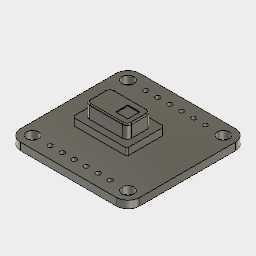
3538 AMG8833 IR Thermal Camera (Autodesk Fusion 360 design; units mm, degrees)
Autodesk Fusion 360 part; units mm, degrees
sketch "AMG8833_REV-B" plane through (0, 0, 0) normal (0, 0, 1) x (1, 0, 0)
  arc A0 (2.54, 25.4) -> (0, 22.86) centre (2.54, 22.86) ccw
  line L0 (2.54, 25.4) -> (22.86, 25.4)
  line L1 (22.86, 0) -> (2.54, 0)
  arc A1 (0, 2.54) -> (2.54, 0) centre (2.54, 2.54) ccw
  line L2 (0, 2.54) -> (0, 22.86)
  arc A2 (22.86, 0) -> (25.4, 2.54) centre (22.86, 2.54) ccw
  arc A3 (25.4, 22.86) -> (22.86, 25.4) centre (22.86, 22.86) ccw
  line L3 (25.4, 22.86) -> (25.4, 2.54)
  circle A4 centre (2.54, 22.86) radius 1.758
  circle A5 centre (8.89, 2.54) radius 0.889
  circle A6 centre (2.54, 22.86) radius 1.758
  circle A7 centre (11.43, 2.54) radius 0.889
  circle A8 centre (22.86, 22.86) radius 1.758
  circle A9 centre (22.86, 2.54) radius 1.758
  circle A10 centre (6.35, 2.54) radius 0.889
  circle A11 centre (22.86, 2.54) radius 1.758
  circle A12 centre (11.43, 2.54) radius 0.889
  circle A13 centre (16.51, 22.86) radius 0.889
  circle A14 centre (13.97, 22.86) radius 0.889
  circle A15 centre (6.35, 22.86) radius 0.889
  circle A16 centre (6.35, 22.86) radius 0.889
  circle A17 centre (2.54, 2.54) radius 1.758
  circle A18 centre (19.05, 22.86) radius 0.889
  circle A19 centre (8.89, 22.86) radius 0.889
  circle A20 centre (11.43, 22.86) radius 0.889
  circle A21 centre (11.43, 22.86) radius 0.889
  circle A22 centre (13.97, 2.54) radius 0.889
  circle A23 centre (16.51, 2.54) radius 0.889
  circle A24 centre (16.51, 2.54) radius 0.889
  circle A25 centre (19.05, 22.86) radius 0.889
  circle A26 centre (16.51, 22.86) radius 0.889
  circle A27 centre (13.97, 22.86) radius 0.889
  circle A28 centre (8.89, 22.86) radius 0.889
  circle A29 centre (6.35, 2.54) radius 0.889
  circle A30 centre (19.05, 2.54) radius 0.889
  circle A31 centre (8.89, 2.54) radius 0.889
  circle A32 centre (13.97, 2.54) radius 0.889
  circle A33 centre (22.86, 22.86) radius 1.758
  circle A34 centre (2.54, 2.54) radius 1.758
  circle A35 centre (19.05, 2.54) radius 0.889
extrude "Extrude2" add sketch "AMG8833_REV-B" along normal blind 1.6
sketch "holes" plane through (0, 0, 1.6) normal (0, 0, 1) x (-1, 0, 0)
  circle A0 centre (-19.05, -2.54) radius 0.889
  circle A1 centre (-6.35, -22.86) radius 0.889
  circle A2 centre (-2.54, -2.54) radius 1.758
  circle A3 centre (-13.97, -22.86) radius 0.889
  circle A4 centre (-19.05, -22.86) radius 0.889
  circle A5 centre (-22.86, -2.54) radius 1.758
  circle A6 centre (-22.86, -22.86) radius 1.758
  circle A7 centre (-6.35, -2.54) radius 0.889
  circle A8 centre (-16.51, -2.54) radius 0.889
  circle A9 centre (-2.54, -22.86) radius 1.758
  circle A10 centre (-13.97, -2.54) radius 0.889
  circle A11 centre (-8.89, -2.54) radius 0.889
  circle A12 centre (-8.89, -22.86) radius 0.889
  circle A13 centre (-11.43, -22.86) radius 0.889
  circle A14 centre (-11.43, -2.54) radius 0.889
  circle A15 centre (-16.51, -22.86) radius 0.889
  arc A16 (-2.54, -25.4) -> (0, -22.86) centre (-2.54, -22.86) ccw
  line L0 (0, -22.86) -> (0, -2.54)
  arc A17 (0, -2.54) -> (-2.54, 0) centre (-2.54, -2.54) ccw
  line L1 (-2.54, 0) -> (-22.86, 0)
  arc A18 (-22.86, 0) -> (-25.4, -2.54) centre (-22.86, -2.54) ccw
  line L2 (-25.4, -2.54) -> (-25.4, -22.86)
  arc A19 (-25.4, -22.86) -> (-22.86, -25.4) centre (-22.86, -22.86) ccw
  line L3 (-22.86, -25.4) -> (-2.54, -25.4)
  circle A20 centre (-22.86, -22.86) radius 1.27
  circle A21 centre (-2.54, -22.86) radius 1.27
  circle A22 centre (-2.54, -2.54) radius 1.27
  circle A23 centre (-22.86, -2.54) radius 1.27
  circle A24 centre (-19.05, -2.54) radius 0.5
  circle A25 centre (-16.51, -2.54) radius 0.5
  circle A26 centre (-13.97, -2.54) radius 0.5
  circle A27 centre (-11.43, -2.54) radius 0.5
  circle A28 centre (-8.89, -2.54) radius 0.5
  circle A29 centre (-6.35, -2.54) radius 0.5
  circle A30 centre (-19.05, -22.86) radius 0.5
  circle A31 centre (-16.51, -22.86) radius 0.5
  circle A32 centre (-13.97, -22.86) radius 0.5
  circle A33 centre (-11.43, -22.86) radius 0.5
  circle A34 centre (-8.89, -22.86) radius 0.5
  circle A35 centre (-6.35, -22.86) radius 0.5
  dimension "d5" = 2.54
  dimension "d6" = 2.54
  dimension "d7" = 2.54
  dimension "d8" = 2.54
  dimension "d9" = 1
  dimension "d15" = 2.54
  dimension "d16" = 0
  dimension "d17" = 1
  dimension "d20" = 2.54
  dimension "d21" = 0
  measures "d5" diameter of A20
  measures "d6" diameter of A21
  measures "d7" diameter of A22
  measures "d8" diameter of A23
  measures "d9" diameter of A24
  measures "d17" diameter of A30
extrude "Extrude3" add sketch "holes" against normal blind 1.6 contours A0 | A1 | A2 | A3 | A4 | A5 | A6 | A7 | A8 | A9 | A10 | A11 | A12 | A13 | A14 | A15
sketch "lens base" plane through (0, 0, 1.6) normal (0, 0, 1) x (-1, 0, 0)
  circle A0 centre (-22.86, -2.54) radius 1.27
  circle A1 centre (-11.43, -2.54) radius 0.5
  circle A2 centre (-22.86, -22.86) radius 1.27
  circle A3 centre (-11.43, -22.86) radius 0.5
  circle A4 centre (-2.54, -22.86) radius 1.27
  circle A5 centre (-13.97, -22.86) radius 0.5
  circle A6 centre (-2.54, -2.54) radius 1.27
  circle A7 centre (-13.97, -2.54) radius 0.5
  circle A8 centre (-19.05, -2.54) radius 0.5
  circle A9 centre (-8.89, -2.54) radius 0.5
  circle A10 centre (-19.05, -22.86) radius 0.5
  circle A11 centre (-8.89, -22.86) radius 0.5
  circle A12 centre (-6.35, -22.86) radius 0.5
  circle A13 centre (-16.51, -22.86) radius 0.5
  circle A14 centre (-6.35, -2.54) radius 0.5
  circle A15 centre (-16.51, -2.54) radius 0.5
  arc A16 (-2.54, -25.4) -> (0, -22.86) centre (-2.54, -22.86) ccw
  line L0 (0, -22.86) -> (0, -2.54)
  arc A17 (0, -2.54) -> (-2.54, 0) centre (-2.54, -2.54) ccw
  line L1 (-2.54, 0) -> (-22.86, 0)
  arc A18 (-22.86, 0) -> (-25.4, -2.54) centre (-22.86, -2.54) ccw
  line L2 (-25.4, -2.54) -> (-25.4, -22.86)
  arc A19 (-25.4, -22.86) -> (-22.86, -25.4) centre (-22.86, -22.86) ccw
  line L3 (-22.86, -25.4) -> (-2.54, -25.4)
  line L4 (-4.868, -16.7) -> (-16.468, -16.7)
  line L5 (-16.468, -16.7) -> (-16.468, -8.7)
  line L6 (-16.468, -8.7) -> (-4.868, -8.7)
  line L7 (-4.868, -8.7) -> (-4.868, -16.7)
  line L8 (-10.668, -16.7) -> (-10.668, -8.7) construction
  line L9 (-16.468, -12.7) -> (-4.868, -12.7) construction
  dimension "d24" = 11.6
  dimension "d25" = 8
  dimension "d26" = 10.668
  dimension "d27" = 12.7
  measures "d24" distance of L4.start L4.end
  measures "d25" distance of L4.start L6.end
  measures "d26" distance of L0 L8
  measures "d27" distance of L1 L9
extrude "Extrude4" add sketch "lens base" along normal blind 1.5 contours L4 L5 L6 L7
sketch "lens" plane through (0, 0, 3.1) normal (0, 0, 1) x (-1, 0, 0)
  line L0 (-4.868, -8.7) -> (-16.468, -8.7)
  line L1 (-16.468, -8.7) -> (-16.468, -16.7)
  line L2 (-16.468, -16.7) -> (-4.868, -16.7)
  line L3 (-4.868, -16.7) -> (-4.868, -8.7)
  line L4 (-11.368, -14) -> (-13.968, -14)
  line L5 (-13.968, -14) -> (-13.968, -11.4)
  line L6 (-13.968, -11.4) -> (-11.368, -11.4)
  line L7 (-11.368, -11.4) -> (-11.368, -14)
  line L8 (-11.368, -12.7) -> (-13.968, -12.7) construction
  line L9 (-12.668, -14) -> (-12.668, -11.4) construction
  line L10 (-10.668, -16.7) -> (-10.668, -8.7) construction
  line L11 (-4.868, -12.7) -> (-16.468, -12.7) construction
  line L12 (-6.218, -15.35) -> (-15.118, -15.35)
  line L13 (-15.118, -15.35) -> (-15.118, -10.05)
  line L14 (-15.118, -10.05) -> (-6.218, -10.05)
  line L15 (-6.218, -10.05) -> (-6.218, -15.35)
  line L16 (-10.668, -15.35) -> (-10.668, -10.05) construction
  line L17 (-6.218, -12.7) -> (-15.118, -12.7) construction
  dimension "d30" = 2.6
  dimension "d31" = 2.6
  dimension "d32" = 2
  dimension "d33" = 8.9
  dimension "d34" = 5.3
  measures "d30" distance of L4.start L4.end
  measures "d31" distance of L4.start L6.end
  measures "d32" distance of L9 L10
  measures "d33" distance of L12.start L12.end
  measures "d34" distance of L12.start L14.end
extrude "Extrude5" add sketch "lens" along normal blind 2.8 contours L4 L5 L6 L7 | L12 L13 L14 L15
fillet "Fillet1" radius 1 4 edges at (6.218, 10.05, 4.5) (6.218, 15.35, 4.5) (15.118, 10.05, 4.5) (15.118, 15.35, 4.5)
fillet "Fillet2" radius 0.25 8 edges at (6.5109, 15.0571, 5.9) (6.218, 12.7, 5.9) (6.5109, 10.3429, 5.9) (10.668, 10.05, 5.9) (14.8251, 10.3429, 5.9) (15.118, 12.7, 5.9) (14.8251, 15.0571, 5.9) (10.668, 15.35, 5.9)
chamfer "Chamfer1" distance 0.4 angle 45 4 edges at (4.868, 16.7, 2.35) (4.868, 8.7, 2.35) (16.468, 16.7, 2.35) (16.468, 8.7, 2.35)
extrude "Extrude6" cut sketch "lens" against normal blind 0.2 from surface at 2.8 contours L4 L5 L6 L7
